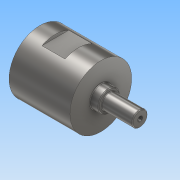
# Autodesk Inventor part: Top_Lever Shaft
Saved by Autodesk Inventor 2018.1 (Build 221171000, 171)
## iProperties
Created: 2019-03-23
Part Number: Top_Lever Shaft
Material: Stainless Steel
Document SubType Name: Modeling
Designer: James
Density: 8 g/cm^3
Appearance: Semi-Polished
Author: James
Autodesk Inventor part; units mm, degrees
ref_plane "YZ Plane" through (0, 0, 0) normal (1, 0, 0) x (0, 1, 0)
ref_plane "XZ Plane" through (0, 0, 0) normal (0, 1, 0) x (-1, 0, 0)
ref_plane "XY Plane" through (0, 0, 0) normal (0, 0, 1) x (1, 0, 0)
sketch "Sketch1" plane through (0, 0, 0) normal (0, 0, 1) x (1, 0, 0)
  line L0 (0, 0) -> (5.5, 0)
  line L1 (5.5, 0) -> (5.5, 7)
  line L2 (5.5, 7) -> (0, 7)
  line L3 (0, 7) -> (0, 0)
  line L4 (5.5, 0) -> (25.5, 0)
  line L5 (25.5, 0) -> (25.5, 5)
  line L6 (25.5, 5) -> (5.5, 5)
  line L7 (5.5, 5) -> (5.5, 0)
  line L8 (0, 0) -> (-39.5, 0)
  line L9 (-39.5, 0) -> (-39.5, 20)
  line L10 (-39.5, 20) -> (0, 20)
  line L11 (0, 20) -> (0, 0)
  dimension "d0" = 5.5
  dimension "d1" = 7
  dimension "d2" = 5
  dimension "d3" = 20
  dimension "d5" = 39.5
  dimension "d6" = 20
  constraints: 24 end point, 6 parallel, 3 horizontal, 3 perpendicular
  measures "d0" distance of L1.end L2.end
  measures "d1" distance between parallel lines of L0 L2
  measures "d2" distance between parallel lines of L4 L6
  measures "d3" distance of L5.end L6.end
  measures "d5" distance of L9.end L10.end
  measures "d6" distance of L8.end L9.end
revolve "Revolution1" add sketch "Sketch1" angle 360 about axis through (5.5, 0, 0) along (1, 0, 0)
sketch "Sketch2" plane through (25.5, 0, 0) normal (1, 0, 0) x (0, 0, -1)
  point P0 (0, 0)
  point P1 (0, 0)
  constraints: 1 coincident
hole "Hole1" at (25.5, 0, 0) direction (-1, 0, 0) diameter 3.242 depth 11.8 tip angle 118 thread size "M4x0.7" class "6H" standard "ANSI Metric M Profile"
sketch "Sketch3" plane through (-39.5, 0, 0) normal (-1, 0, 0) x (0, 0, 1)
  point P0 (0, 0)
  point P1 (0, 0)
  constraints: 1 coincident
hole "Hole2" at (-39.5, 0, 0) direction (1, 0, 0) diameter 6.647 depth 22.2 tip angle 118 thread size "M8x1.25" class "6H" standard "ANSI Metric M Profile"
sketch "Sketch4" plane through (0, 0, 0) normal (0, 1, 0) x (-1, 0, 0)
  line L0 (29.5, -20) -> (14.5, -20)
  line L1 (14.5, -20) -> (14.5, -18)
  line L2 (14.5, -18) -> (29.5, -18)
  line L3 (29.5, -18) -> (29.5, -20)
  line L4 (14.5, 20) -> (29.5, 20)
  line L5 (29.5, 20) -> (29.5, 18)
  line L6 (29.5, 18) -> (14.5, 18)
  line L7 (14.5, 18) -> (14.5, 20)
  line L8 (39.5, 20) -> (39.5, -20) projected
  point P0 (0, 0)
  dimension "d21" = 15
  dimension "d22" = 36
  dimension "d23" = 2
  dimension "d24" = 2
  dimension "d25" = 10
  constraints: 16 end point, 4 parallel, 2 horizontal, 2 horizontal alignment, 2 perpendicular, 2 vertical alignment, 1 point on line
  measures "d21" distance of L0.start L0.end
  measures "d22" distance between parallel lines of L6 L2
  measures "d23" distance from line of L8.end L2
  measures "d24" distance between parallel lines of L4 L6
  measures "d25" distance between parallel lines of L3 L8
extrude "Extrusion1" cut sketch "Sketch4" along normal through all both and the other way through all
fillet "Fillet1" radius 0.5 1 edges at (0, -7, 0)
fillet "Fillet2" radius 0.4 1 edges at (5.5, -5, 0)
chamfer "Chamfer1" distance 0.5 angle 45 1 edges at (25.5, -5, 0)
chamfer "Chamfer2" distance 0.5 angle 45 1 edges at (5.5, -7, 0)
equation "\"d23\" = d24"
body "Solid1"
